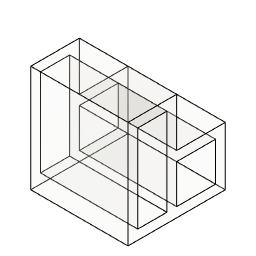
stepToMilz (Autodesk Fusion 360 design; units mm, degrees)
Autodesk Fusion 360 part; units mm, degrees
sketch "Sketch1" plane through (0, 0, 0) normal (0, 0, 1) x (1, 0, 0)
  line L0 (32.3278, 26.7056) -> (232.3278, 26.7056)
  line L1 (232.3278, 26.7056) -> (232.3278, 226.7056)
  line L2 (232.3278, 226.7056) -> (32.3278, 226.7056)
  line L3 (32.3278, 226.7056) -> (32.3278, 26.7056)
  dimension "d1" = 200
  dimension "d2" = 200
  constraint horizontal L0
  constraint vertical L1
  constraint horizontal L2
  constraint vertical L3
  measures "d1" distance of L0.start L0.end
  measures "d2" distance of L0.start L2.end
extrude "Extrude1" add sketch "Sketch1" along normal blind 20
sketch "Sketch2" plane through (0, 0, 20) normal (0, 0, 1) x (-1, 0, 0)
  line L0 (-32.3278, -226.7056) -> (-32.3278, -26.7056)
  line L1 (-32.3278, -26.7056) -> (-232.3278, -26.7056)
  line L2 (-232.3278, -26.7056) -> (-232.3278, -226.7056)
  line L3 (-232.3278, -226.7056) -> (-32.3278, -226.7056)
  line L4 (-232.3278, -226.7056) -> (-32.3278, -226.7056)
  line L5 (-32.3278, -226.7056) -> (-32.3278, -206.7056)
  line L6 (-32.3278, -206.7056) -> (-232.3278, -206.7056)
  line L7 (-232.3278, -206.7056) -> (-232.3278, -226.7056)
  dimension "d5" = 20
  constraint horizontal L4
  constraint vertical L5
  constraint horizontal L6
  constraint vertical L7
  constraint coincident L2.end L3.start
  measures "d5" distance of L2.end L6.end
extrude "Extrude2" add sketch "Sketch2" along normal blind 100 contours L0 L2 L3 L4 L5 L6 L7
sketch "Sketch3" plane through (0, 206.7056, 0) normal (0, -1, 0) x (1, 0, 0)
  line L0 (32.3278, 20) -> (232.3278, 20)
  line L1 (232.3278, 20) -> (232.3278, 120)
  line L2 (232.3278, 120) -> (32.3278, 120)
  line L3 (32.3278, 120) -> (32.3278, 20)
  line L4 (32.3278, 120) -> (232.3278, 120)
  line L5 (232.3278, 120) -> (232.3278, 100)
  line L6 (232.3278, 100) -> (32.3278, 100)
  line L7 (32.3278, 100) -> (32.3278, 120)
  dimension "d8" = 200
  dimension "d9" = 20
  constraint horizontal L4
  constraint vertical L5
  constraint horizontal L6
  constraint vertical L7
  constraint coincident L2.end L3.start
  measures "d8" distance of L2.end L1.end
  measures "d9" distance of L2.end L6.end
extrude "Extrude3" add sketch "Sketch3" along normal blind 80 contours L1 L2 L3 L4 L5 L6 L7
sketch "Sketch4" plane through (0, 0, 20) normal (0, 0, 1) x (-1, 0, 0)
  line L0 (-232.3278, -206.7056) -> (-32.3278, -206.7056)
  line L1 (-32.3278, -206.7056) -> (-32.3278, -26.7056)
  line L2 (-32.3278, -26.7056) -> (-232.3278, -26.7056)
  line L3 (-232.3278, -26.7056) -> (-232.3278, -206.7056)
  line L4 (-232.3278, -26.7056) -> (-32.3278, -26.7056)
  line L5 (-32.3278, -26.7056) -> (-32.3278, -46.7056)
  line L6 (-32.3278, -46.7056) -> (-232.3278, -46.7056)
  line L7 (-232.3278, -46.7056) -> (-232.3278, -26.7056)
  line L8 (-232.3278, -26.7056) -> (-232.3278, -106.7056)
  line L9 (-232.3278, -106.7056) -> (-32.3278, -106.7056)
  line L10 (-32.3278, -106.7056) -> (-32.3278, -126.7056)
  line L11 (-32.3278, -126.7056) -> (-232.3278, -126.7056)
  line L12 (-232.3278, -126.7056) -> (-232.3278, -106.7056)
  dimension "d12" = 20
  dimension "d13" = 80
  dimension "d14" = 20
  constraint horizontal L4
  constraint vertical L5
  constraint horizontal L6
  constraint vertical L7
  constraint coincident L2.end L3.start
  constraint perpendicular L0 L8
  constraint horizontal L9
  constraint vertical L10
  constraint horizontal L11
  constraint vertical L12
  measures "d12" distance of L2.end L6.end
  measures "d13" distance of L2.end L8.end
  measures "d14" distance of L8.end L11.end
extrude "Extrude4" add sketch "Sketch4" along normal blind 200 contours L1 L3 L9 L10 L11 L12 | L1 L2 L3 L4 L5 L6 L7 L8
sketch "Sketch5" plane through (0, 46.7056, 0) normal (0, 1, 0) x (-1, 0, 0)
  line L0 (-232.3278, 20) -> (-32.3278, 20)
  line L1 (-32.3278, 20) -> (-32.3278, 220)
  line L2 (-32.3278, 220) -> (-232.3278, 220)
  line L3 (-232.3278, 220) -> (-232.3278, 20)
  line L4 (-232.3278, 220) -> (-32.3278, 220)
  line L5 (-32.3278, 220) -> (-32.3278, 200)
  line L6 (-32.3278, 200) -> (-232.3278, 200)
  line L7 (-232.3278, 200) -> (-232.3278, 220)
  dimension "d17" = 20
  constraint horizontal L4
  constraint vertical L5
  constraint horizontal L6
  constraint vertical L7
  constraint coincident L2.end L3.start
  measures "d17" distance of L2.end L6.end
extrude "Extrude5" add sketch "Sketch5" along normal blind 60 contours L1 L2 L3 L4 L5 L6 L7
